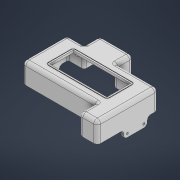
# Autodesk Inventor part: Cover Shield
Saved by Autodesk Inventor 2021 (Build 250183000, 183)
## iProperties
Created: 2025-01-15
Part Number: Cover Shield
Material: Generic
Document SubType Name: Modeling
Designer: user
Density: 1 g/cm^3
Appearance: Default
Author: user
## iProperties of the stored document _3DPrint.ipt
Created: 2025-01-15
Part Number: _3DPrint
Material: Generic
Document SubType Name: Modeling
Designer: user
Density: 1 g/cm^3
Appearance: Default
Author: user
Autodesk Inventor part; units mm, degrees
ref_plane "YZ Plane" through (0, 0, 0) normal (1, 0, 0) x (0, 1, 0)
ref_plane "XZ Plane" through (0, 0, 0) normal (0, 1, 0) x (-1, 0, 0)
ref_plane "XY Plane" through (0, 0, 0) normal (0, 0, 1) x (1, 0, 0)
sketch "Sketch1" plane through (0, 0, 0) normal (0, 1, 0) x (-1, 0, 0)
  line L0 (141.8339, -117.4498) -> (0, -117.4498)
  line L1 (141.8339, -114.7981) -> (141.8339, -117.4498)
  line L2 (141.8339, 0) -> (141.8339, -114.7727)
  line L3 (141.8339, -114.7981) -> (141.8339, -114.7727)
  circle A0 centre (139.8146, -115.4305) radius 1.016
  circle A1 centre (2.5273, -115.0495) radius 1.016
  line L4 (0, -117.4498) -> (0, 0)
  line L5 (0, 0) -> (141.8339, 0)
  circle A2 centre (2.4003, -2.4003) radius 1.016
  circle A3 centre (139.8146, -2.0193) radius 1.016
  line L6 (136.9296, -111.2815) -> (136.9296, -109.2815)
  line L7 (119.8396, -99.4815) -> (119.8396, -97.4815)
  line L8 (136.9296, -111.2815) -> (119.8396, -111.2815)
  line L9 (119.8396, -111.2815) -> (119.8396, -97.4815)
  line L10 (119.8396, -97.4815) -> (136.9296, -97.4815)
  line L11 (136.9296, -97.4815) -> (136.9296, -111.2815)
  line L12 (61.8724, -111.2815) -> (61.8724, -109.2815)
  line L13 (6.4283, -99.7355) -> (6.4283, -97.7355)
  line L14 (61.8724, -111.2815) -> (6.4283, -111.2815)
  line L15 (6.4283, -111.2815) -> (6.4283, -97.7355)
  line L16 (6.4283, -97.7355) -> (61.8724, -97.7355)
  line L17 (61.8724, -97.7355) -> (61.8724, -111.2815)
  line L18 (137.7026, -8.0933) -> (137.7026, -7.5933)
  line L19 (137.6026, -7.4933) -> (135.5026, -7.4933)
  line L20 (25.3134, -20.4213) -> (27.4134, -20.4213)
  line L21 (25.2134, -19.8213) -> (25.2134, -20.3213)
  line L22 (25.2134, -20.4213) -> (137.7026, -20.4213)
  line L23 (137.7026, -20.4213) -> (137.7026, -7.4933)
  line L24 (137.7026, -7.4933) -> (25.2134, -7.4933)
  line L25 (25.2134, -7.4933) -> (25.2134, -20.4213)
  line L26 (-1, -118.4498) -> (142.8339, -118.4498)
  line L27 (142.8339, -118.4498) -> (142.8339, -114.7981)
  line L28 (142.8339, -114.7981) -> (142.8339, -114.7727)
  line L29 (142.8339, -114.7727) -> (142.8339, 1)
  line L30 (142.8339, 1) -> (-1, 1)
  line L31 (-1, 1) -> (-1, -118.4498)
  line L32 (141.8339, -123.4498) -> (0, -123.4498)
  line L33 (-6, -117.4498) -> (-6, 0)
  line L34 (0, 6) -> (141.8339, 6)
  line L35 (147.8339, 0) -> (147.8339, -114.7727)
  line L36 (147.8339, -114.7727) -> (147.8339, -114.7981)
  line L37 (147.8339, -114.7981) -> (147.8339, -117.4498)
  circle A4 centre (139.8146, -115.4305) radius 1.4
  circle A5 centre (2.5273, -115.0495) radius 1.4
  circle A6 centre (2.4003, -2.4003) radius 1.4
  circle A7 centre (139.8146, -2.0193) radius 1.4
  circle A8 centre (139.8146, -115.4305) radius 4.4
  circle A9 centre (2.5273, -115.0495) radius 4.4
  circle A10 centre (2.4003, -2.4003) radius 4.4
  circle A11 centre (139.8146, -2.0193) radius 4.4
  arc A12 (141.8339, -123.4498) -> (147.8339, -117.4498) centre (141.8339, -117.4498) ccw
  arc A13 (-6, -117.4498) -> (0, -123.4498) centre (0, -117.4498) ccw
  arc A14 (0, 6) -> (-6, 0) centre (0, 0) ccw
  arc A15 (147.8339, 0) -> (141.8339, 6) centre (141.8339, 0) ccw
  line L38 (64.8724, -123.4498) -> (118.8396, -123.4498)
  line L39 (111.8396, -118.4498) -> (69.8724, -118.4498)
  line L40 (-6, -21.4213) -> (147.8339, -21.4213)
  line L41 (-6, -96.7355) -> (147.8339, -96.7355)
  line L42 (-6, -24.4213) -> (147.8339, -24.4213)
  line L43 (-6, -93.7355) -> (147.8339, -93.7355)
  line L44 (62.8724, -93.7355) -> (118.8396, -93.7355)
  line L45 (118.8396, -93.7355) -> (118.8396, -123.4498)
  line L46 (118.8396, -123.4498) -> (62.8724, -123.4498)
  line L47 (62.8724, -123.4498) -> (62.8724, -93.7355)
  line L48 (65.8724, -96.7355) -> (115.8396, -96.7355)
  line L49 (115.8396, -93.7355) -> (115.8396, -118.4498)
  line L50 (65.8724, -118.4498) -> (65.8724, -93.7355)
  line L51 (24.2134, -24.4213) -> (24.2134, 6)
  line L52 (21.2134, -24.4213) -> (21.2134, 6)
  point P0 (136.614, 1)
  point P1 (142.8339, -5.2199)
  point P2 (136.614, -118.4498)
  point P3 (142.8339, -112.2299)
  point P4 (5.3198, -118.4498)
  point P5 (-1, -112.4193)
  point P6 (-1, -5.1928)
  point P7 (5.1928, 1)
  point P8 (128.3846, -97.4815)
  point P9 (24.2134, -21.4213)
  point P10 (-1, -96.7355)
  point P11 (-1, -93.7355)
  point P12 (0, -93.7355)
  point P13 (0, -96.7355)
  point P14 (62.8724, -96.7355)
  point P15 (118.8396, -96.7355)
  point P16 (21.2134, 1)
  point P17 (142.8339, -24.4213)
  point P18 (142.8339, -93.7355)
  dimension "d0" = 1
  dimension "d1" = 5
  dimension "d2" = 2.8
  dimension "d3" = 2.8
  dimension "d4" = 2.8
  dimension "d5" = 2.8
  dimension "d6" = 3
  dimension "d7" = 3
  dimension "d8" = 3
  dimension "d9" = 3
  dimension "d10" = 6
  dimension "d32" = 1
  dimension "d33" = 1
  dimension "d34" = 3
  dimension "d35" = 3
  dimension "d36" = 1
  dimension "d37" = 1
  dimension "d38" = 3
  dimension "d39" = 1
  dimension "d40" = 3
  constraints: 106 end point, 16 centre point, 14 point on line, 12 parallel, 8 horizontal, 8 point on circle, 8 tangent, 7 perpendicular, 5 vertical, 4 coincident, 3 equal radius, 1 midpoint, 11 other
  measures "d0" distance between parallel lines of L0 L26
  measures "d1" distance between parallel lines of L26 L32
  measures "d2" diameter of A4
  measures "d3" diameter of A5
  measures "d4" diameter of A6
  measures "d5" diameter of A7
  measures "d6" radial gap between concentric circles of A4 A8
  measures "d7" radial gap between concentric circles of A5 A9
  measures "d8" radial gap between concentric circles of A6 A10
  measures "d9" radial gap between concentric circles of A7 A11
  measures "d10" radius of A12
  measures "d32" distance between parallel lines of L22 L40
  measures "d33" distance between parallel lines of L41 L16
  measures "d34" distance between parallel lines of L40 L42
  measures "d35" distance between parallel lines of L41 L43
  measures "d36" distance between parallel lines of L17 L47
  measures "d37" distance between parallel lines of L9 L45
  measures "d38" distance between parallel lines of L47 L50
  measures "d39" distance between parallel lines of L25 L51
  measures "d40" distance between parallel lines of L51 L52
extrude "Extrusion4" add sketch "Sketch1" along normal blind 4 contours L45 L26 L49 L0 | L0 L49 L41 L45 | L49 L26 L50 L0 | L0 L50 L41 L49 | L45 L43 L2 L41 | L41 L49 L43 L45 | L45 L32 L47 L26 | L2 L43 L29 L41 | L50 L26 L47 L0 | L0 L47 L41 L50 | L41 L50 L43 L49 | L43 L4 L42 L2 | L2 L42 L29 L43 | L29 L43 L35 L41 | L41 L47 L43 L50 | L42 L51 L40 L2 | L2 L40 L29 L42 | L29 L42 L35 L43 | L41 L4 L43 L47 | L42 L52 L40 L51 | L29 L40 L35 L42 | L41 L31 L43 L4 | L40 L52 L5 L51 | L42 L4 L40 L52 | L43 L31 L42 L4 | L41 L33 L43 L31 | L40 L4 A10 L5 L52 | L5 L52 L30 L51 | L42 L31 L40 L4 | L43 L33 L42 L31 | L40 L31 A10 L4 | L5 A10 L30 L52 | L30 L52 L34 L51 | L42 L33 L40 L31 | A10 L31 L30 L5 L4 | L4 L5 A10 | L40 L33 A14 L34 L52 L30 A10 L31 | A10 L31 | L30 A10 | L31 L30 A10 | A2 | A6
extrude "Extrusion5" add sketch "Sketch1" against normal blind 30 contours L45 L26 L49 L0 | L0 L49 L41 L45 | L45 L43 L2 L41 | L41 L49 L43 L45 | L45 L32 L47 L26 | L2 L43 L29 L41 | L50 L26 L47 L0 | L0 L47 L41 L50 | L29 L43 L35 L41 | L41 L47 L43 L50 | L42 L51 L40 L2 | L2 L40 L29 L42 | L29 L42 L35 L43 | L41 L4 L43 L47 | L42 L52 L40 L51 | L29 L40 L35 L42 | L41 L31 L43 L4 | L40 L52 L5 L51 | L41 L33 L43 L31 | L5 L52 L30 L51 | L43 L33 L42 L31 | L30 L52 L34 L51 | L42 L33 L40 L31 | L40 L33 A14 L34 L52 L30 A10 L31 | A10 L31 | L30 A10
fillet "Fillet3" radius 6 6 edges at (-62.8724, -13, -123.4498) (-118.8396, -13, -123.4498) (-147.8339, -13, -96.7355) (-147.8339, -13, -21.4213) (6, -13, -96.7355) (-24.2134, -13, 6)
fillet "Fillet3" radius 1 3 edges at (-24.2134, -13, -21.4213) (-62.8724, -13, -96.7355) (-118.8396, -13, -96.7355)
fillet "Fillet3" radius 3 5 edges at (-142.8339, -15, -24.4213) (-142.8339, -15, -93.7355) (1, -15, -93.7355) (1, -15, 1) (-21.2134, -15, 1)
fillet "Fillet3" radius 4 3 edges at (-65.8724, -15, -93.7355) (-115.8396, -15, -93.7355) (-21.2134, -15, -24.4213)
fillet "Fillet4" radius 2 17 edges at (-141.9552, 0, -25.3) (-142.8339, 0, -59.0784) (-141.9552, 0, -92.8568) (-129.8367, 0, -93.7355) (-117.0111, 0, -94.9071) (-115.8396, 0, -108.0927) (-22.3849, 0, -23.2498) (-21.2134, 0, -11.2107) (-20.3347, 0, 0.1213) (-10.1067, 0, 1) (0.1213, 0, 0.1213) (1, 0, -46.3678) (0.1213, 0, -92.8568) (-31.9362, 0, -93.7355) (-64.7008, 0, -94.9071) (-65.8724, 0, -108.0927) (-82.5236, 0, -24.4213)
fillet "Fillet4" radius 6 20 edges at (4.2426, 4, -94.9782) (-30.9362, 4, -96.7355) (-62.5795, 4, -97.0284) (-62.8724, 4, -107.5927) (-64.6298, 4, -121.6925) (-90.856, 4, -123.4498) (-117.0822, 4, -121.6925) (-118.8396, 4, -107.5927) (-119.1325, 4, -97.0284) (-130.8367, 4, -96.7355) (-146.0765, 4, -94.9782) (-147.8339, 4, -59.0784) (-146.0765, 4, -23.1787) (-83.5236, 4, -21.4213) (-24.5063, 4, -21.1285) (-24.2134, 4, -10.2107) (-22.456, 4, 4.2426) (-9.1067, 4, 6) (4.2426, 4, 4.2426) (6, 4, -45.3678)
sketch "Sketch3" plane through (-147.8339, -30, -90.7355) normal (-1, 0, 0) x (0, 0, 1)
  circle A0 centre (46.0106, -8) radius 1.4 projected
  circle A1 centre (18.0106, -8) radius 1.4 projected
  line L0 (53.5385, -2) -> (10.4827, -2) projected
  arc A2 (12.0106, -6) -> (10.4827, -2) centre (6.0106, -6) ccw projected
  line L1 (12.0106, -8) -> (12.0106, -6) projected
  arc A3 (12.0106, -8) -> (18.0106, -14) centre (18.0106, -8) ccw projected
  line L2 (46.0106, -14) -> (18.0106, -14) projected
  arc A4 (46.0106, -14) -> (52.0106, -8) centre (46.0106, -8) ccw projected
  line L3 (52.0106, -6) -> (52.0106, -8) projected
  arc A5 (53.5385, -2) -> (52.0106, -6) centre (58.0106, -6) ccw projected
  line L4 (63.3142, 0) -> (0, 0) projected
  arc A6 (12.0106, -6) -> (6.0106, 0) centre (6.0106, -6) ccw projected
  arc A7 (58.0106, 0) -> (52.0106, -6) centre (58.0106, -6) ccw projected
  line L5 (51.8106, -6) -> (51.8106, -8)
  arc A8 (46.0106, -13.8) -> (51.8106, -8) centre (46.0106, -8) ccw
  line L6 (46.0106, -13.8) -> (18.0106, -13.8)
  arc A9 (12.2106, -8) -> (18.0106, -13.8) centre (18.0106, -8) ccw
  line L7 (12.2106, -8) -> (12.2106, -6)
  arc A10 (12.2106, -6) -> (10.9096, -2.2) centre (6.0106, -6) ccw
  line L8 (10.9096, -2.2) -> (53.1116, -2.2)
  arc A11 (53.1116, -2.2) -> (51.8106, -6) centre (58.0106, -6) ccw
  arc A12 (12.2106, -6) -> (6.0106, 0.2) centre (6.0106, -6) ccw
  arc A13 (58.0106, 0.2) -> (51.8106, -6) centre (58.0106, -6) ccw
  circle A14 centre (18.0106, -8) radius 1.7
  circle A15 centre (46.0106, -8) radius 1.7
  point P0 (90.7355, 30)
  point P1 (53.1116, -2.2)
  point P2 (56.4485, 0)
  point P3 (7.5726, 0)
  point P4 (10.9096, -2.2)
  point P5 (12.2106, -6)
  dimension "d51" = 0.2
  dimension "d52" = 0.2
  dimension "d53" = 0.2
  dimension "d54" = 0.2
  dimension "d55" = 3.4
  dimension "d56" = 3.4
  constraints: 12 point on circle, 8 centre point, 8 end point, 2 coincident, 6 other
  measures "d51" radial gap between concentric circles of A3 A9
  measures "d52" radial gap between concentric circles of A2 A10
  measures "d53" radial gap between concentric circles of A6 A12
  measures "d54" radial gap between concentric circles of A7 A13
  measures "d55" diameter of A14
  measures "d56" diameter of A15
extrude "Extrusion6" add sketch "Sketch3" against normal blind 5 contours A13 L8 A12 L0 | L0 A12 L4 A13 | A11 L5 A8 L6 A9 L7 A10 L8
sketch "Sketch4" plane through (6, -30, 0) normal (1, 0, 0) x (0, 0, -1)
  circle A0 centre (72.7249, -8) radius 1.7 projected
  circle A1 centre (44.7249, -8) radius 1.7 projected
  line L0 (27.4213, 28) -> (90.7355, 28) projected
  line L1 (27.4213, 0) -> (27.4213, 28) projected
  line L2 (34.287, 0) -> (27.4213, 0) projected
  arc A2 (38.9249, -6) -> (34.287, 0) centre (32.7249, -6) ccw projected
  line L3 (38.9249, -6) -> (38.9249, -8) projected
  arc A3 (38.9249, -8) -> (44.7249, -13.8) centre (44.7249, -8) ccw projected
  line L4 (44.7249, -13.8) -> (72.7249, -13.8) projected
  arc A4 (72.7249, -13.8) -> (78.5249, -8) centre (72.7249, -8) ccw projected
  line L5 (78.5249, -8) -> (78.5249, -6) projected
  arc A5 (83.1629, 0) -> (78.5249, -6) centre (84.7249, -6) ccw projected
  line L6 (90.7355, 0) -> (83.1629, 0) projected
  line L7 (90.7355, 28) -> (90.7355, 0) projected
  line L8 (90.7355, 0) -> (0, 0) projected
  point P0 (0, 30)
extrude "Extrusion7" add sketch "Sketch4" against normal blind 5 contours L8 A5 L5 A4 L4 A3 L3 A2
sketch "Sketch5" plane through (-68.8724, -30, -123.4498) normal (0, 0, -1) x (-1, 0, 0)
  line L0 (43.9672, 0) -> (0, 0) projected
  line L1 (1.9811, 2.1) -> (19.7611, 2.1) projected
  line L2 (14.0785, 16.5346) -> (7.7785, 16.5346)
  arc A0 (7.7785, 16.5346) -> (7.0785, 15.8346) centre (7.7785, 15.8346) ccw
  line L3 (7.0785, 15.8346) -> (7.0785, 15.0361)
  arc A1 (7.0785, 15.0361) -> (7.2835, 14.5411) centre (7.7785, 15.0361) ccw
  line L4 (7.2835, 14.5411) -> (7.5074, 14.3173)
  arc A2 (14.7785, 15.8346) -> (14.0785, 16.5346) centre (14.0785, 15.8346) ccw
  line L5 (14.7785, 15.8346) -> (14.7785, 15.0361)
  arc A3 (14.5735, 14.5411) -> (14.7785, 15.0361) centre (14.0785, 15.0361) ccw
  line L6 (8.3285, 13.9347) -> (13.5285, 13.9347)
  arc A4 (7.5953, 14.1051) -> (7.5074, 14.3173) centre (7.2953, 14.1051) ccw
  line L7 (7.5953, 14.1051) -> (7.5953, 13.3347)
  arc A5 (7.5953, 13.3347) -> (8.2953, 12.6347) centre (8.2953, 13.3347) ccw
  line L8 (8.2953, 12.6347) -> (13.5617, 12.6347)
  arc A6 (13.5617, 12.6347) -> (14.2617, 13.3347) centre (13.5617, 13.3347) ccw
  line L9 (14.2617, 14.1051) -> (14.2617, 13.3347)
  arc A7 (14.3496, 14.3173) -> (14.2617, 14.1051) centre (14.5617, 14.1051) ccw
  line L10 (14.5735, 14.5411) -> (14.3496, 14.3173)
  line L11 (70.9615, 0) -> (-43.659, 0) projected
  line L12 (10.9285, 0) -> (20.9285, 0)
  line L13 (10.9285, 0) -> (10.9285, 12.635)
  line L14 (2.9285, 9.5411) -> (18.9285, 9.5411)
  line L15 (20.9285, 11.5411) -> (20.9285, 17.5411)
  line L16 (18.9285, 19.5411) -> (2.9285, 19.5411)
  line L17 (0.9285, 17.5411) -> (0.9285, 11.5411)
  line L18 (0.9285, 9.5411) -> (20.9285, 19.5411) construction
  line L19 (20.9285, 9.5411) -> (0.9285, 19.5411) construction
  arc A8 (2.9285, 19.5411) -> (0.9285, 17.5411) centre (2.9285, 17.5411) ccw
  arc A9 (20.9285, 17.5411) -> (18.9285, 19.5411) centre (18.9285, 17.5411) ccw
  arc A10 (18.9285, 9.5411) -> (20.9285, 11.5411) centre (18.9285, 11.5411) ccw
  arc A11 (0.9285, 11.5411) -> (2.9285, 9.5411) centre (2.9285, 11.5411) ccw
  point P0 (-68.8724, 30)
  point P1 (10.9285, 13.9347)
  point P2 (10.9285, 12.6347)
  point P3 (10.9285, 14.5411)
  dimension "d61" = 10
  dimension "d62" = 12.635
  dimension "d63" = 20
  dimension "d64" = 10
  dimension "d65" = 2
  constraints: 34 end point, 24 point on circle, 12 centre point, 10 point on line, 8 tangent, 4 midpoint, 3 equal radius, 2 parallel, 2 perpendicular, 1 horizontal
  measures "d61" distance of L12.start L12.end
  measures "d62" distance of L12.start L13.end
  measures "d63" distance of L19.end L18.end
  measures "d64" distance of L18.end L19.start
  measures "d65" radius of A8
extrude "Extrusion8" cut sketch "Sketch5" against normal blind 5 contours A2 L5 A3 L10 A7 L9 A6 L8 A5 L7 A4 L4 A1 L3 A0 L2 | L14 A11 L17 A8 L16 A9 L15 A10
sketch "Sketch6" plane through (0, 4, 0) normal (0, 1, 0) x (1, 0, 0)
  line L0 (-22.6376, 39.0587) -> (-22.6376, 78.7587)
  line L1 (-22.6376, 78.7587) -> (-119.1376, 78.7587)
  line L2 (-119.1376, 78.7587) -> (-119.1376, 39.0587)
  line L3 (-119.1376, 39.0587) -> (-22.6376, 39.0587)
  line L4 (0, 187.124) -> (104.4116, 187.124)
  line L5 (-4.5962, 0) -> (-4.5962, 187.124)
  circle A0 centre (-24.3876, 31.4087) radius 1.5
  circle A1 centre (-24.3876, 86.4087) radius 1.5
  circle A2 centre (-117.3876, 31.4087) radius 1.5
  circle A3 centre (-117.3876, 86.4087) radius 1.5
  line L6 (-118.3876, 79.4087) -> (-23.3876, 79.4087)
  line L7 (-119.8876, 39.9087) -> (-119.8876, 77.9087)
  arc A4 (-118.3876, 79.4087) -> (-119.8876, 77.9087) centre (-118.3876, 77.9087) ccw
  line L8 (-23.3876, 38.4087) -> (-118.3876, 38.4087)
  arc A5 (-23.3876, 38.4087) -> (-21.8876, 39.9087) centre (-23.3876, 39.9087) ccw
  line L9 (-21.8876, 77.9087) -> (-21.8876, 39.9087)
  arc A6 (-21.8876, 77.9087) -> (-23.3876, 79.4087) centre (-23.3876, 77.9087) ccw
  line L10 (-70.8876, 38.4087) -> (-70.8876, 79.4087)
  arc A7 (-119.8876, 39.9087) -> (-118.3876, 38.4087) centre (-118.3876, 39.9087) ccw
  line L11 (-21.8876, 58.9087) -> (-119.8876, 58.9087)
  line L12 (-22.6376, 58.9087) -> (-119.1376, 58.9087)
  line L13 (-70.8876, 39.0587) -> (-70.8876, 78.7587)
  circle A8 centre (-24.3876, 31.4087) radius 1.4
  circle A9 centre (-117.3876, 31.4087) radius 1.4
  circle A10 centre (-117.3876, 86.4087) radius 1.4
  circle A11 centre (-24.3876, 86.4087) radius 1.4
  circle A12 centre (-24.3876, 86.4087) radius 4.4
  circle A13 centre (-24.3876, 31.4087) radius 4.4
  circle A14 centre (-117.3876, 31.4087) radius 4.4
  circle A15 centre (-117.3876, 86.4087) radius 4.4
  line L14 (-22.3376, 79.0587) -> (-22.3376, 38.7587)
  line L15 (-22.3376, 38.7587) -> (-119.4376, 38.7587)
  line L16 (-119.4376, 38.7587) -> (-119.4376, 79.0587)
  line L17 (-119.4376, 79.0587) -> (-22.3376, 79.0587)
  line L18 (-23.3876, 81.4087) -> (-118.3876, 81.4087)
  arc A16 (-118.3876, 81.4087) -> (-121.8876, 77.9087) centre (-118.3876, 77.9087) ccw
  line L19 (-121.8876, 77.9087) -> (-121.8876, 39.9087)
  arc A17 (-121.8876, 39.9087) -> (-118.3876, 36.4087) centre (-118.3876, 39.9087) ccw
  line L20 (-118.3876, 36.4087) -> (-23.3876, 36.4087)
  arc A18 (-23.3876, 36.4087) -> (-19.8876, 39.9087) centre (-23.3876, 39.9087) ccw
  line L21 (-19.8876, 39.9087) -> (-19.8876, 77.9087)
  arc A19 (-19.8876, 77.9087) -> (-23.3876, 81.4087) centre (-23.3876, 77.9087) ccw
  line L22 (-118.3876, 82.4087) -> (-23.3876, 82.4087)
  arc A20 (-18.8876, 77.9087) -> (-23.3876, 82.4087) centre (-23.3876, 77.9087) ccw
  line L23 (-18.8876, 77.9087) -> (-18.8876, 39.9087)
  arc A21 (-23.3876, 35.4087) -> (-18.8876, 39.9087) centre (-23.3876, 39.9087) ccw
  line L24 (-23.3876, 35.4087) -> (-118.3876, 35.4087)
  arc A22 (-122.8876, 39.9087) -> (-118.3876, 35.4087) centre (-118.3876, 39.9087) ccw
  line L25 (-122.8876, 39.9087) -> (-122.8876, 77.9087)
  arc A23 (-118.3876, 82.4087) -> (-122.8876, 77.9087) centre (-118.3876, 77.9087) ccw
  point P0 (0, 0)
  point P1 (0, 0)
  point P2 (-16, 0)
  point P3 (52.2058, 187.124)
  point P4 (-4.5962, 93.562)
  point P5 (-119.8876, 28.9087)
  point P6 (-70.8876, 58.9087)
  point P7 (-70.8876, 58.9087)
  dimension "d68" = 39.7
  dimension "d69" = 96.5
  dimension "d70" = 2.8
  dimension "d71" = 2.8
  dimension "d72" = 2.8
  dimension "d73" = 2.8
  dimension "d74" = 3
  dimension "d75" = 3
  dimension "d76" = 3
  dimension "d77" = 3
  dimension "d78" = 0.3
  dimension "d83" = 2
  dimension "d84" = 1
  constraints: 52 end point, 24 centre point, 24 point on circle, 12 midpoint, 4 coincident, 4 parallel, 2 perpendicular, 17 other
  measures "d68" distance of L2.end L1.end
  measures "d69" distance of L1.end L0.end
  measures "d70" diameter of A8
  measures "d71" diameter of A9
  measures "d72" diameter of A10
  measures "d73" diameter of A11
  measures "d74" radial gap between concentric circles of A11 A12
  measures "d75" radial gap between concentric circles of A8 A13
  measures "d76" radial gap between concentric circles of A9 A14
  measures "d77" radial gap between concentric circles of A10 A15
  measures "d78" distance between parallel lines of L0 L14
  measures "d83" distance between parallel lines of L6 L18
  measures "d84" distance between parallel lines of L18 L22
extrude "Extrusion9" cut sketch "Sketch6" against normal blind 5 contours L3 L10 L11 L0 | L0 L11 L14 A5 L15 L10 L3 | L11 L10 L1 L0 | L0 L1 L10 L17 A6 L14 L11 | L10 L15 A7 L16 L11 L2 L3 | L3 L2 L11 L10 | L11 L2 L1 L10 | L1 L2 L11 L16 A4 L17 L10 | A6 L17 L14 | L14 L15 A5 | L15 L16 A7 | A4 L16 L17
extrude "Extrusion10" add sketch "Sketch6" against normal blind 9 contours A0 | A1 | A2 | A3 | A12 A20 L22 | L22 A20 A12 | L22 A23 A15 | A15 A23 L22 | A21 L24 A13 | A13 L24 A21 | A22 L24 A14 | A14 L24 A22
extrude "Extrusion11" cut sketch "Sketch6" against normal blind 0.6 contours L22 A20 A12 | A12 A20 L23 A21 A13 L24 A14 A22 L25 A23 A15 L22 | A15 A23 L22 | A21 L24 A13 | A14 L24 A22 picked at (-24.9892, 82.3116) picked at (-116.786, 82.3116) picked at (-24.9892, 35.5058) picked at (-116.786, 35.5058)
body "Solid2"
